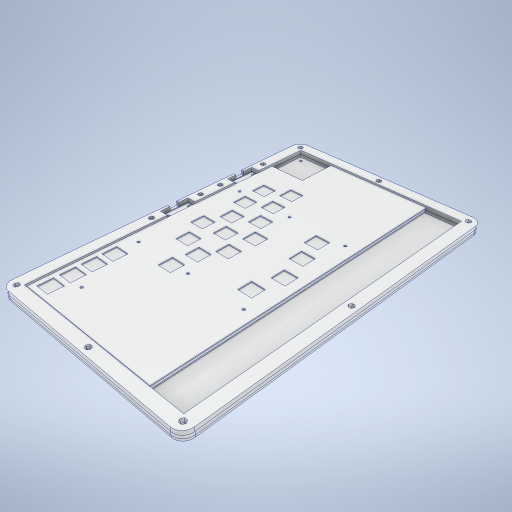
# Autodesk Inventor part: frame
Saved by Autodesk Inventor 2024 (Build 280153000, 153)
## iProperties
Created: 2023-10-23
Part Number: frame
Material: 铝 6061
Document SubType Name: Modeling
Designer: nicx5
Density: 2.7 g/cm^3
Appearance: 铝 - 平面
Author: nicx5
Autodesk Inventor part; units mm, degrees
ref_plane "YZ Plane" through (0, 0, 0) normal (1, 0, 0) x (0, 1, 0)
ref_plane "XY Plane" through (0, 0, 0) normal (0, 0, 1) x (1, 0, 0)
ref_plane "FloorFirst平面" through (0, 2, 0) normal (0, 1, 0) x (-1, 0, 0)
ref_plane "FloorSecond平面" through (0, 5, 0) normal (0, 1, 0) x (-1, 0, 0)
ref_plane "TopPlate平面" through (0, 9, 0) normal (0, 1, 0) x (-1, 0, 0)
ref_plane "PCB平面" through (0, 3.8, 0) normal (0, 1, 0) x (-1, 0, 0)
ref_plane "PositionPlate平面" through (0, 7, 0) normal (0, 1, 0) x (-1, 0, 0)
sketch "OLED草图" plane through (0, 0, 0) normal (0, 1, 0) x (-1, 0, 0)
  line L0 (84.9998, -145.0002) -> (84.9998, -109.6002)
  line L1 (84.9998, -109.6002) -> (51.4998, -109.6002)
  line L2 (51.4998, -145.0002) -> (84.9998, -145.0002)
  line L3 (51.4998, -109.6002) -> (51.4998, -145.0002)
  circle A0 centre (82.4998, -112.2002) radius 1.5
  circle A1 centre (82.4998, -142.4002) radius 1.5
  circle A2 centre (53.9998, -112.2002) radius 1.5
  circle A3 centre (53.9998, -142.4002) radius 1.5
  line L4 (61.9498, -111.5902) -> (61.9498, -143.0102)
  line L5 (61.9498, -143.0102) -> (78.6498, -143.0102)
  line L6 (78.6498, -143.0102) -> (78.6498, -111.5902)
  line L7 (78.6498, -111.5902) -> (61.9498, -111.5902)
  line L8 (84.9998, -115.8002) -> (78.6498, -115.8002)
  line L9 (78.6498, -115.8002) -> (78.6498, -138.8002)
  line L10 (78.6498, -138.8002) -> (84.9998, -138.8002)
  line L11 (84.9998, -138.8002) -> (84.9998, -115.8002)
  point P0 (0, 0)
  constraints: 24 end point, 4 centre point
sketch "BottomPlate草图" plane through (0, 0, 0) normal (0, 1, 0) x (-1, 0, 0)
  line L0 (90, 160) -> (-90, 160)
  line L1 (-100, 150) -> (-100, -150)
  line L2 (-90, -160) -> (90, -160)
  line L3 (100, -150) -> (100, 150)
  line L4 (-100, 160) -> (100, -160) construction
  circle A0 centre (92, 152) radius 1.6
  circle A1 centre (92, -152) radius 1.6
  circle A2 centre (-92, 152) radius 1.6
  circle A3 centre (-92, -152) radius 1.6
  arc A4 (100, 150) -> (90, 160) centre (90, 150) ccw
  arc A5 (-90, 160) -> (-100, 150) centre (-90, 150) ccw
  arc A6 (-100, -150) -> (-90, -160) centre (-90, -150) ccw
  arc A7 (90, -160) -> (100, -150) centre (90, -150) ccw
  circle A8 centre (94, 26.75) radius 2.75
  circle A9 centre (94, -26.75) radius 2.75
  circle A10 centre (94, -49.75) radius 2.75
  circle A11 centre (94, -103.25) radius 2.75
  circle A12 centre (0, 154) radius 2.75
  circle A13 centre (0, -153.5) radius 2.75
  circle A14 centre (-94, 0) radius 2.75
  circle A15 centre (91.5, 11) radius 1.35
  circle A16 centre (91.5, -11) radius 1.35
  circle A17 centre (91.5, -65.5) radius 1.35
  circle A18 centre (91.5, -87.5) radius 1.35
  circle A19 centre (16, 55) radius 1.35
  circle A20 centre (16, -55) radius 1.35
  circle A21 centre (75, 55) radius 1.35
  circle A22 centre (75, -55) radius 1.35
  circle A23 centre (57.5, 120) radius 1.35
  circle A24 centre (-43, 55) radius 1.35
  circle A25 centre (-43, -55) radius 1.35
  circle A26 centre (82.4998, -112.2002) radius 1.5 projected
  circle A27 centre (82.4998, -142.4002) radius 1.5 projected
  circle A28 centre (53.9998, -142.4002) radius 1.5 projected
  circle A29 centre (53.9998, -112.2002) radius 1.5 projected
  dimension "d12" = 3.2
  dimension "d13" = 3.2
  dimension "d14" = 3.2
  dimension "d15" = 3.2
  dimension "d16" = 10
  dimension "d58" = 5.5
  dimension "d59" = 5.5
  dimension "d60" = 5.5
  dimension "d61" = 5.5
  dimension "d63" = 5.5
  dimension "d65" = 5.5
  dimension "d67" = 5.5
  dimension "d210" = 2.7
  dimension "d211" = 2.7
  dimension "d214" = 2.7
  dimension "d215" = 2.7
  dimension "d218" = 2.7
  dimension "d219" = 2.7
  dimension "d227" = 2.7
  dimension "d228" = 2.7
  dimension "d237" = 2.7
  dimension "d325" = 2.7
  dimension "d326" = 2.7
  constraints: 26 centre point, 10 end point, 8 point on circle, 8 tangent, 4 point on line, 3 equal radius
  measures "d12" diameter of A0
  measures "d13" diameter of A1
  measures "d14" diameter of A2
  measures "d15" diameter of A3
  measures "d16" radius of A4
  measures "d58" diameter of A8
  measures "d59" diameter of A9
  measures "d60" diameter of A10
  measures "d61" diameter of A11
  measures "d63" diameter of A12
  measures "d65" diameter of A13
  measures "d67" diameter of A14
  measures "d210" diameter of A15
  measures "d211" diameter of A16
  measures "d214" diameter of A17
  measures "d215" diameter of A18
  measures "d218" diameter of A19
  measures "d219" diameter of A20
  measures "d227" diameter of A21
  measures "d228" diameter of A22
  measures "d237" diameter of A23
  measures "d325" diameter of A24
  measures "d326" diameter of A25
sketch "FloorFirst草图" plane through (0, 2, 0) normal (0, 1, 0) x (-1, 0, 0)
  arc A0 (100, 150) -> (90, 160) centre (90, 150) ccw
  line L0 (100, -150) -> (100, 150)
  arc A1 (90, -160) -> (100, -150) centre (90, -150) ccw
  line L1 (-90, -160) -> (90, -160)
  arc A2 (-100, -150) -> (-90, -160) centre (-90, -150) ccw
  line L2 (-100, 150) -> (-100, -150)
  arc A3 (-90, 160) -> (-100, 150) centre (-90, 150) ccw
  line L3 (90, 160) -> (-90, 160)
  circle A4 centre (-92, 152) radius 1.6
  line L4 (89.2557, 152) -> (90.6279, 154.3766)
  line L5 (90.6279, 154.3766) -> (93.3721, 154.3766)
  line L6 (93.3721, 154.3766) -> (94.7443, 152)
  line L7 (94.7443, 152) -> (93.3721, 149.6234)
  line L8 (93.3721, 149.6234) -> (90.6279, 149.6234)
  line L9 (90.6279, 149.6234) -> (89.2557, 152)
  line L10 (-94.7495, 152) -> (-93.3747, 154.3811)
  line L11 (-93.3747, 154.3811) -> (-90.6253, 154.3811)
  line L12 (-90.6253, 154.3811) -> (-89.2505, 152)
  line L13 (-89.2505, 152) -> (-90.6253, 149.6189)
  line L14 (-90.6253, 149.6189) -> (-93.3747, 149.6189)
  line L15 (-93.3747, 149.6189) -> (-94.7495, 152)
  line L16 (-94.7495, -152) -> (-93.3747, -149.6189)
  line L17 (-93.3747, -149.6189) -> (-90.6253, -149.6189)
  line L18 (-90.6253, -149.6189) -> (-89.2505, -152)
  line L19 (-89.2505, -152) -> (-90.6253, -154.3811)
  line L20 (-90.6253, -154.3811) -> (-93.3747, -154.3811)
  line L21 (-93.3747, -154.3811) -> (-94.7495, -152)
  line L22 (89.2506, -152) -> (90.6253, -149.6189)
  line L23 (90.6253, -149.6189) -> (93.3747, -149.6189)
  line L24 (93.3747, -149.6189) -> (94.7494, -152)
  line L25 (94.7494, -152) -> (93.3747, -154.3811)
  line L26 (93.3747, -154.3811) -> (90.6253, -154.3811)
  line L27 (90.6253, -154.3811) -> (89.2506, -152)
  line L28 (88, 148) -> (-88, 148)
  line L29 (-88, 148) -> (-88, -148)
  line L30 (-88, -148) -> (88, -148)
  line L31 (97, -15) -> (97, 15)
  line L32 (97, -15) -> (97, -4.9)
  line L33 (88, -15) -> (97, -15)
  line L34 (97, 15) -> (88, 15)
  line L35 (97, -61.5) -> (97, -91.5)
  line L36 (97, -81.4) -> (97, -91.5)
  line L37 (97, -91.5) -> (88, -91.5)
  line L38 (88, -61.5) -> (97, -61.5)
  line L39 (88, 15) -> (88, 148)
  line L40 (88, -148) -> (88, -91.5)
  line L41 (88, -61.5) -> (88, -15)
  line L42 (91.25, 26.75) -> (92.625, 29.1316)
  line L43 (92.625, 29.1316) -> (95.375, 29.1316)
  line L44 (95.375, 29.1316) -> (96.75, 26.75)
  line L45 (96.75, 26.75) -> (95.375, 24.3684)
  line L46 (95.375, 24.3684) -> (92.625, 24.3684)
  line L47 (92.625, 24.3684) -> (91.25, 26.75)
  line L48 (91.25, -26.75) -> (92.625, -24.3684)
  line L49 (92.625, -24.3684) -> (95.375, -24.3684)
  line L50 (95.375, -24.3684) -> (96.75, -26.75)
  line L51 (96.75, -26.75) -> (95.375, -29.1316)
  line L52 (95.375, -29.1316) -> (92.625, -29.1316)
  line L53 (92.625, -29.1316) -> (91.25, -26.75)
  line L54 (91.25, -49.75) -> (92.625, -47.3684)
  line L55 (92.625, -47.3684) -> (95.375, -47.3684)
  line L56 (95.375, -47.3684) -> (96.75, -49.75)
  line L57 (96.75, -49.75) -> (95.375, -52.1316)
  line L58 (95.375, -52.1316) -> (92.625, -52.1316)
  line L59 (92.625, -52.1316) -> (91.25, -49.75)
  line L60 (91.25, -103.25) -> (92.625, -100.8684)
  line L61 (92.625, -100.8684) -> (95.375, -100.8684)
  line L62 (95.375, -100.8684) -> (96.75, -103.25)
  line L63 (96.75, -103.25) -> (95.375, -105.6316)
  line L64 (95.375, -105.6316) -> (92.625, -105.6316)
  line L65 (92.625, -105.6316) -> (91.25, -103.25)
  line L66 (-2.7499, 154) -> (-1.375, 156.3815)
  line L67 (-1.375, 156.3815) -> (1.375, 156.3815)
  line L68 (1.375, 156.3815) -> (2.7499, 154)
  line L69 (2.7499, 154) -> (1.375, 151.6185)
  line L70 (1.375, 151.6185) -> (-1.375, 151.6185)
  line L71 (-1.375, 151.6185) -> (-2.7499, 154)
  line L72 (-2.7499, -153.5) -> (-1.375, -151.1185)
  line L73 (-1.375, -151.1185) -> (1.375, -151.1185)
  line L74 (1.375, -151.1185) -> (2.7499, -153.5)
  line L75 (2.7499, -153.5) -> (1.375, -155.8815)
  line L76 (1.375, -155.8815) -> (-1.375, -155.8815)
  line L77 (-1.375, -155.8815) -> (-2.7499, -153.5)
  line L78 (-96.75, 0) -> (-95.375, 2.3816)
  line L79 (-95.375, 2.3816) -> (-92.625, 2.3816)
  line L80 (-92.625, 2.3816) -> (-91.25, 0)
  line L81 (-91.25, 0) -> (-92.625, -2.3816)
  line L82 (-92.625, -2.3816) -> (-95.375, -2.3816)
  line L83 (-95.375, -2.3816) -> (-96.75, 0)
  point P0 (0, 0)
  point P1 (92, 152)
  point P2 (-92, -152)
  point P3 (92, -152)
  point P4 (94, 26.75)
  point P5 (94, -26.75)
  point P6 (94, -49.75)
  point P7 (94, -103.25)
  point P8 (0, 154)
  point P9 (0, -153.5)
  point P10 (-94, 0)
  constraints: 168 end point, 8 point on circle, 5 centre point, 145 other
sketch "FloorSecond草图" plane through (0, 5, 0) normal (0, 1, 0) x (-1, 0, 0)
  arc A0 (100, 150) -> (90, 160) centre (90, 150) ccw
  line L0 (90, 160) -> (-90, 160)
  arc A1 (-90, 160) -> (-100, 150) centre (-90, 150) ccw
  line L1 (-100, 150) -> (-100, -150)
  arc A2 (-100, -150) -> (-90, -160) centre (-90, -150) ccw
  line L2 (-90, -160) -> (90, -160)
  arc A3 (90, -160) -> (100, -150) centre (90, -150) ccw
  line L3 (88, 148) -> (-88, 148)
  line L4 (-88, 148) -> (-88, -148)
  line L5 (-88, -148) -> (88, -148)
  line L6 (94.7443, 152) -> (93.3721, 149.6234)
  line L7 (93.3721, 154.3766) -> (94.7443, 152)
  line L8 (90.6279, 154.3766) -> (93.3721, 154.3766)
  line L9 (89.2557, 152) -> (90.6279, 154.3766)
  line L10 (90.6279, 149.6234) -> (89.2557, 152)
  line L11 (93.3721, 149.6234) -> (90.6279, 149.6234)
  line L12 (90.6253, -149.6189) -> (93.3747, -149.6189)
  line L13 (93.3747, -149.6189) -> (94.7494, -152)
  line L14 (94.7494, -152) -> (93.3747, -154.3811)
  line L15 (93.3747, -154.3811) -> (90.6253, -154.3811)
  line L16 (90.6253, -154.3811) -> (89.2506, -152)
  line L17 (89.2506, -152) -> (90.6253, -149.6189)
  line L18 (-89.2505, -152) -> (-90.6253, -154.3811)
  line L19 (-90.6253, -149.6189) -> (-89.2505, -152)
  line L20 (-93.3747, -149.6189) -> (-90.6253, -149.6189)
  line L21 (-94.7495, -152) -> (-93.3747, -149.6189)
  line L22 (-93.3747, -154.3811) -> (-94.7495, -152)
  line L23 (-90.6253, -154.3811) -> (-93.3747, -154.3811)
  line L24 (-90.6253, 154.3811) -> (-89.2505, 152)
  line L25 (-93.3747, 154.3811) -> (-90.6253, 154.3811)
  line L26 (-94.7495, 152) -> (-93.3747, 154.3811)
  line L27 (-93.3747, 149.6189) -> (-94.7495, 152)
  line L28 (-90.6253, 149.6189) -> (-93.3747, 149.6189)
  line L29 (-89.2505, 152) -> (-90.6253, 149.6189)
  line L30 (97, 15) -> (88, 15)
  line L31 (88, -15) -> (97, -15)
  line L32 (88, 15) -> (88, 148)
  line L33 (100, 4.9) -> (97, 4.9)
  line L34 (97, -4.9) -> (100, -4.9)
  line L35 (97, -15) -> (97, -4.9)
  line L36 (97, 4.9) -> (97, 15)
  line L37 (88, -15) -> (93, -15)
  line L38 (93, -61.5) -> (88, -61.5)
  line L39 (88, -61.5) -> (88, -15)
  line L40 (88, -61.5) -> (97, -61.5)
  line L41 (97, -91.5) -> (88, -91.5)
  line L42 (100, -71.6) -> (97, -71.6)
  line L43 (97, -81.4) -> (100, -81.4)
  line L44 (97, -61.5) -> (97, -71.6)
  line L45 (97, -81.4) -> (97, -91.5)
  line L46 (100, 4.9) -> (100, 150)
  line L47 (100, -150) -> (100, -81.4)
  line L48 (100, -71.6) -> (100, -4.9)
  line L49 (88, -148) -> (88, -91.5)
  line L50 (88, -61.5) -> (88, -15)
  line L51 (96.75, 26.75) -> (95.375, 24.3684)
  line L52 (95.375, 29.1316) -> (96.75, 26.75)
  line L53 (92.625, 29.1316) -> (95.375, 29.1316)
  line L54 (91.25, 26.75) -> (92.625, 29.1316)
  line L55 (92.625, 24.3684) -> (91.25, 26.75)
  line L56 (95.375, 24.3684) -> (92.625, 24.3684)
  line L57 (96.75, -26.75) -> (95.375, -29.1316)
  line L58 (95.375, -24.3684) -> (96.75, -26.75)
  line L59 (92.625, -24.3684) -> (95.375, -24.3684)
  line L60 (91.25, -26.75) -> (92.625, -24.3684)
  line L61 (92.625, -29.1316) -> (91.25, -26.75)
  line L62 (95.375, -29.1316) -> (92.625, -29.1316)
  line L63 (95.375, -47.3684) -> (96.75, -49.75)
  line L64 (92.625, -47.3684) -> (95.375, -47.3684)
  line L65 (91.25, -49.75) -> (92.625, -47.3684)
  line L66 (92.625, -52.1316) -> (91.25, -49.75)
  line L67 (95.375, -52.1316) -> (92.625, -52.1316)
  line L68 (96.75, -49.75) -> (95.375, -52.1316)
  line L69 (95.375, -100.8684) -> (96.75, -103.25)
  line L70 (92.625, -100.8684) -> (95.375, -100.8684)
  line L71 (91.25, -103.25) -> (92.625, -100.8684)
  line L72 (92.625, -105.6316) -> (91.25, -103.25)
  line L73 (95.375, -105.6316) -> (92.625, -105.6316)
  line L74 (96.75, -103.25) -> (95.375, -105.6316)
  line L75 (2.7499, -153.5) -> (1.375, -155.8815)
  line L76 (1.375, -151.1185) -> (2.7499, -153.5)
  line L77 (-1.375, -151.1185) -> (1.375, -151.1185)
  line L78 (-2.7499, -153.5) -> (-1.375, -151.1185)
  line L79 (-1.375, -155.8815) -> (-2.7499, -153.5)
  line L80 (1.375, -155.8815) -> (-1.375, -155.8815)
  line L81 (-91.25, 0) -> (-92.625, -2.3816)
  line L82 (-92.625, 2.3816) -> (-91.25, 0)
  line L83 (-95.375, 2.3816) -> (-92.625, 2.3816)
  line L84 (-96.75, 0) -> (-95.375, 2.3816)
  line L85 (-95.375, -2.3816) -> (-96.75, 0)
  line L86 (-92.625, -2.3816) -> (-95.375, -2.3816)
  line L87 (1.375, 156.3815) -> (2.7499, 154)
  line L88 (-1.375, 156.3815) -> (1.375, 156.3815)
  line L89 (-2.7499, 154) -> (-1.375, 156.3815)
  line L90 (-1.375, 151.6185) -> (-2.7499, 154)
  line L91 (1.375, 151.6185) -> (-1.375, 151.6185)
  line L92 (2.7499, 154) -> (1.375, 151.6185)
  point P0 (0, 0)
  point P1 (88, 0)
  point P2 (97, 0)
  point P3 (97, -76.5)
  constraints: 186 end point, 8 point on circle, 4 centre point
sketch "TopPlate草图" plane through (0, 9, 0) normal (0, 1, 0) x (-1, 0, 0)
  line L0 (100, 4.9) -> (100, 150)
  arc A0 (100, 150) -> (90, 160) centre (90, 150) ccw
  line L1 (90, 160) -> (-90, 160)
  line L2 (100, -150) -> (100, 150)
  arc A1 (90, -160) -> (100, -150) centre (90, -150) ccw
  line L3 (-90, -160) -> (90, -160)
  arc A2 (-100, -150) -> (-90, -160) centre (-90, -150) ccw
  line L4 (-100, 150) -> (-100, -150)
  arc A3 (-90, 160) -> (-100, 150) centre (-90, 150) ccw
  circle A4 centre (92, 152) radius 1.6
  circle A5 centre (92, -152) radius 1.6
  circle A6 centre (-92, -152) radius 1.6
  circle A7 centre (-92, 152) radius 1.6
  line L5 (32.0321, 53.8512) -> (32.0321, 31.8512) construction
  arc A8 (15.4226, 25.1627) -> (25.9869, 17.7656) centre (15.5932, 14.1641) ccw
  line L6 (28.2118, 32.1854) -> (28.2118, 10.1854) construction
  circle A9 centre (13.4288, -12.5738) radius 11
  circle A10 centre (-30.7795, 35.3233) radius 11
  line L7 (-30.7795, 35.3233) -> (-37.9769, 8.2642)
  line L8 (-37.9769, 8.2642) -> (-30.7795, -18.795)
  circle A11 centre (-37.9769, 8.2642) radius 13.5
  circle A12 centre (-30.7795, -18.795) radius 11
  line L9 (13.4288, -12.5738) -> (-10.8955, -12.5738) construction
  line L10 (13.4288, -12.5738) -> (-18.1395, -12.5738) construction
  line L11 (13.4288, -12.5738) -> (-18.1395, -12.5738) construction
  line L12 (13.4288, -12.5738) -> (27.7683, -33.0526)
  line L13 (13.4288, -12.5738) -> (-11.5712, -12.5738) construction
  line L14 (27.7683, -33.0526) -> (36.3188, -56.5449)
  line L15 (36.3188, -56.5449) -> (38.4977, -81.4497)
  line L16 (15.5932, 14.1641) -> (29.0722, 33.4141)
  line L17 (15.5932, 14.1641) -> (-7.9068, 14.1641) construction
  line L18 (29.0722, 33.4141) -> (33.1529, 56.5571)
  circle A13 centre (27.7683, -33.0526) radius 11
  circle A14 centre (36.3188, -56.5449) radius 11
  circle A15 centre (38.4977, -81.4497) radius 11
  line L19 (58.7471, -45.803) -> (60.926, -70.7079)
  circle A16 centre (60.926, -70.7079) radius 11
  circle A17 centre (58.7471, -45.803) radius 11
  circle A18 centre (35.8572, -1.8319) radius 11
  circle A19 centre (50.1966, -22.3107) radius 11
  line L20 (50.1966, -22.3107) -> (58.7471, -45.803)
  line L21 (35.8572, -1.8319) -> (50.1966, -22.3107)
  circle A20 centre (60.7621, 0.347) radius 11
  line L22 (-30.7795, -18.795) -> (-24.4131, -42.9707)
  circle A21 centre (-24.4131, -42.9707) radius 11
  line L23 (36.0371, 44.12) -> (36.0361, 44.1148)
  line L24 (26.43, 20.9234) -> (26.4269, 20.919)
  line L25 (26.189, 45.8565) -> (26.1881, 45.8512)
  line L26 (18.2384, 26.6592) -> (18.2354, 26.6548)
  arc A22 (37.9557, 46.661) -> (25.2551, 48.9005) centre (33.1529, 56.5571) ccw
  arc A23 (24.2694, 43.3102) -> (18.6785, 29.8126) centre (29.0722, 33.4141) ccw
  arc A24 (37.9557, 46.661) -> (36.0371, 44.12) centre (39.4839, 43.5122) ccw
  arc A25 (36.0361, 44.1148) -> (36.97, 41.0708) centre (39.483, 43.507) ccw
  arc A26 (26.189, 45.8565) -> (25.2551, 48.9005) centre (22.7422, 46.4642) ccw
  arc A27 (24.2694, 43.3102) -> (26.1881, 45.8512) centre (22.7412, 46.459) ccw
  arc A28 (29.2427, 22.4155) -> (26.43, 20.9234) centre (29.297, 18.9159) ccw
  arc A29 (26.4269, 20.919) -> (25.9869, 17.7656) centre (29.2939, 18.9115) ccw
  arc A30 (18.2384, 26.6592) -> (18.6785, 29.8126) centre (15.3714, 28.6667) ccw
  arc A31 (15.4226, 25.1627) -> (18.2354, 26.6548) centre (15.3684, 28.6623) ccw
  line L27 (85, 145) -> (64.7, 145)
  line L28 (64.7, 145) -> (64.7, 67.7)
  line L29 (64.7, 67.7) -> (85, 67.7)
  line L30 (85, 67.7) -> (85, 145)
  line L31 (74.85, 134.85) -> (74.85, 115.85)
  line L32 (74.85, 115.85) -> (74.85, 96.85)
  line L33 (74.85, 96.85) -> (74.85, 77.85)
  line L34 (29.0722, 33.4141) -> (50.7834, 24.4211)
  line L35 (29.0722, 33.4141) -> (52.5722, 33.4141) construction
  arc A32 (40.0823, 21.874) -> (45.0176, 33.7889) centre (50.7834, 24.4211) ccw
  arc A33 (29.2427, 22.4155) -> (34.838, 24.0463) centre (29.0722, 33.4141) ccw
  arc A34 (39.7733, 35.9612) -> (36.97, 41.0708) centre (29.0722, 33.4141) ccw
  line L36 (38.0168, 24.2972) -> (38.0119, 24.2992)
  line L37 (41.8437, 33.536) -> (41.8387, 33.538)
  arc A35 (40.0823, 21.874) -> (38.0168, 24.2972) centre (36.6774, 21.0636) ccw
  arc A36 (38.0119, 24.2992) -> (34.838, 24.0463) centre (36.6725, 21.0656) ccw
  arc A37 (41.8437, 33.536) -> (45.0176, 33.7889) centre (43.1831, 36.7696) ccw
  arc A38 (39.7733, 35.9612) -> (41.8387, 33.538) centre (43.1781, 36.7716) ccw
  line L38 (84.9998, -109.6002) -> (51.4998, -109.6002)
  line L39 (51.4998, -109.6002) -> (51.4998, -145.0002)
  line L40 (51.4998, -145.0002) -> (84.9998, -145.0002)
  line L41 (84.9998, -145.0002) -> (84.9998, -109.6002)
  line L42 (84.9998, -115.8002) -> (78.6498, -115.8002)
  line L43 (78.6498, -115.8002) -> (78.6498, -138.8002)
  line L44 (78.6498, -138.8002) -> (84.9998, -138.8002)
  line L45 (84.9998, -138.8002) -> (84.9998, -115.8002)
  line L46 (78.6498, -111.5902) -> (61.9498, -111.5902)
  line L47 (61.9498, -111.5902) -> (61.9498, -143.0102)
  line L48 (61.9498, -143.0102) -> (78.6498, -143.0102)
  line L49 (78.6498, -143.0102) -> (78.6498, -111.5902)
  line L50 (84.9998, -109.6002) -> (82.4998, -109.6002)
  line L51 (82.4998, -109.6002) -> (82.4998, -112.2002)
  line L52 (82.4998, -112.2002) -> (84.9998, -112.2002)
  line L53 (84.9998, -112.2002) -> (84.9998, -109.6002)
  line L54 (84.9998, -145.0002) -> (82.4998, -145.0002)
  line L55 (82.4998, -145.0002) -> (82.4998, -142.4002)
  line L56 (82.4998, -142.4002) -> (84.9998, -142.4002)
  line L57 (84.9998, -142.4002) -> (84.9998, -145.0002)
  line L58 (51.4998, -109.6002) -> (53.9998, -109.6002)
  line L59 (53.9998, -109.6002) -> (53.9998, -112.2002)
  line L60 (53.9998, -112.2002) -> (51.4998, -112.2002)
  line L61 (51.4998, -112.2002) -> (51.4998, -109.6002)
  line L62 (51.4998, -145.0002) -> (53.9998, -145.0002)
  line L63 (53.9998, -145.0002) -> (53.9998, -142.4002)
  line L64 (53.9998, -142.4002) -> (51.4998, -142.4002)
  line L65 (51.4998, -142.4002) -> (51.4998, -145.0002)
  circle A39 centre (82.4998, -112.2002) radius 1.5
  circle A40 centre (82.4998, -142.4002) radius 1.5
  circle A41 centre (53.9998, -142.4002) radius 1.5
  circle A42 centre (53.9998, -112.2002) radius 1.5
  circle A43 centre (92, 152) radius 1.6 projected
  circle A44 centre (0, 154) radius 2.75 projected
  circle A45 centre (-92, 152) radius 1.6 projected
  circle A46 centre (-94, 0) radius 2.75 projected
  circle A47 centre (-92, -152) radius 1.6 projected
  circle A48 centre (0, -153.5) radius 2.75 projected
  circle A49 centre (92, -152) radius 1.6 projected
  circle A50 centre (94, 26.75) radius 2.75 projected
  circle A51 centre (94, -26.75) radius 2.75 projected
  point P0 (33.9026, 43.7117)
  point P1 (36.3756, 46.0398)
  point P2 (27.5481, 22.5202)
  point P3 (26.5275, 47.7762)
  point P4 (17.1173, 25.058)
  point P5 (35.6976, 42.195)
  point P6 (25.8496, 43.9315)
  point P7 (19.3566, 28.256)
  point P8 (25.3088, 19.3222)
  point P9 (39.8178, 23.5512)
  point P10 (43.6447, 32.79)
  point P11 (36.2109, 25.0452)
  point P12 (40.0378, 34.284)
  dimension "d102" = 22
  dimension "d103" = 22
  dimension "d104" = 27
  dimension "d105" = 22
  dimension "d106" = 22
  dimension "d107" = 25
  dimension "d108" = 125
  dimension "d109" = 25
  dimension "d110" = 165
  dimension "d111" = 25
  dimension "d112" = 165
  dimension "d113" = 23.5
  dimension "d114" = 125
  dimension "d115" = 23.5
  dimension "d116" = 155
  dimension "d117" = 22
  dimension "d118" = 22
  dimension "d119" = 22
  dimension "d120" = 22
  dimension "d121" = 25
  dimension "d122" = 25
  dimension "d123" = 165
  dimension "d124" = 25
  dimension "d125" = 165
  dimension "d126" = 22
  dimension "d127" = 22
  dimension "d128" = 22
  dimension "d129" = 22
  dimension "d130" = 25
  dimension "d131" = 22
  dimension "d134" = 5
  dimension "d135" = 5
  dimension "d136" = 3.5
  dimension "d137" = 3.5
  dimension "d138" = 3.5
  dimension "d139" = 3.5
  dimension "d142" = 20.3
  dimension "d143" = 77.3
  dimension "d145" = 19
  dimension "d146" = 19
  dimension "d147" = 19
  dimension "d169" = 23.5
  dimension "d170" = 22.5
  dimension "d171" = 22
  dimension "d174" = 3.5
  dimension "d175" = 3.5
  dimension "d180" = 33.5
  dimension "d181" = 35.4
  dimension "d183" = 6.35
  dimension "d184" = 23
  dimension "d186" = 16.7
  dimension "d187" = 31.42
  dimension "d188" = 2.5
  dimension "d189" = 2.6
  dimension "d190" = 2.5
  dimension "d191" = 2.6
  dimension "d192" = 2.5
  dimension "d193" = 2.6
  dimension "d194" = 2.5
  dimension "d195" = 2.6
  dimension "d196" = 3
  dimension "d197" = 3
  dimension "d198" = 3
  dimension "d199" = 3
  constraints: 132 end point, 54 point on circle, 43 centre point, 22 tangent, 13 point on line, 8 coincident, 6 equal radius, 3 equal length, 1 horizontal, 1 parallel
  measures "d102" diameter of A8
  measures "d103" diameter of A9
  measures "d104" diameter of A11
  measures "d105" diameter of A10
  measures "d106" diameter of A12
  measures "d107" distance of L12.start L12.end
  measures "d108" angle of L13 L12
  measures "d109" distance of L12.end L14.end
  measures "d110" angle of L12 L14
  measures "d111" distance of L14.end L15.end
  measures "d112" angle of L14 L15
  measures "d113" distance of L16.start L16.end
  measures "d114" angle of L16 L17
  measures "d115" distance of L16.end L18.end
  measures "d116" angle of L18 L16
  measures "d117" diameter of A13
  measures "d118" diameter of A14
  measures "d119" diameter of A15
  measures "d120" diameter of A18
  measures "d121" distance of L21.start L21.end
  measures "d122" distance of L21.end L20.end
  measures "d123" angle of L21 L20
  measures "d124" distance of L20.end L19.end
  measures "d125" angle of L20 L19
  measures "d126" diameter of A19
  measures "d127" diameter of A17
  measures "d128" diameter of A16
  measures "d129" diameter of A20
  measures "d130" distance of L22.start L22.end
  measures "d131" diameter of A21
  measures "d134" distance between parallel lines of L18 L23
  measures "d135" distance between parallel lines of L18 L25
  measures "d136" radius of A24
  measures "d137" radius of A26
  measures "d138" radius of A27
  measures "d139" radius of A28
  measures "d142" distance of L29.end L28.end
  measures "d143" distance of L28.end L27.end
  measures "d145" distance of L31.start L31.end
  measures "d146" distance of L32.start L32.end
  measures "d147" distance of L33.start L33.end
  measures "d169" distance of L34.start L34.end
  measures "d170" angle of L34 L35
  measures "d171" diameter of A32
  measures "d174" radius of A35
  measures "d175" radius of A37
  measures "d180" distance of L40.end L39.end
  measures "d181" distance of L39.end L38.end
  measures "d183" distance of L44.end L43.end
  measures "d184" distance of L43.end L42.end
  measures "d186" distance of L48.end L47.end
  measures "d187" distance of L47.end L46.end
  measures "d188" distance of L52.end L51.end
  measures "d189" distance of L51.end L50.end
  measures "d190" distance of L55.end L56.end
  measures "d191" distance of L54.end L55.end
  measures "d192" distance of L59.end L60.end
  measures "d193" distance of L58.end L59.end
  measures "d194" distance of L64.end L63.end
  measures "d195" distance of L63.end L62.end
  measures "d196" diameter of A39
  measures "d197" diameter of A40
  measures "d198" diameter of A41
  measures "d199" diameter of A42
sketch "PositionPlate草图" plane through (0, 7, 0) normal (0, 1, 0) x (-1, 0, 0)
  line L0 (87, 147) -> (87, -107.6002)
  line L1 (87, -90.5) -> (87, -147)
  line L2 (49.4998, -147) -> (-54.9998, -147)
  line L3 (-54.9998, -147) -> (-54.9998, 147)
  line L4 (-54.9998, 147) -> (87, 147)
  line L5 (74.85, 134.85) -> (74.85, 115.85) projected
  line L6 (74.85, 115.85) -> (74.85, 96.85) projected
  line L7 (74.85, 96.85) -> (74.85, 77.85) projected
  line L8 (29.0722, 33.4141) -> (50.7834, 24.4211) projected
  line L9 (29.0722, 33.4141) -> (33.1529, 56.5571) projected
  line L10 (15.5932, 14.1641) -> (29.0722, 33.4141) projected
  line L11 (35.8572, -1.8319) -> (50.1966, -22.3107) projected
  line L12 (50.1966, -22.3107) -> (58.7471, -45.803) projected
  line L13 (58.7471, -45.803) -> (60.926, -70.7079) projected
  line L14 (13.4288, -12.5738) -> (27.7683, -33.0526) projected
  line L15 (27.7683, -33.0526) -> (36.3188, -56.5449) projected
  line L16 (36.3188, -56.5449) -> (38.4977, -81.4497) projected
  line L17 (-30.7795, 35.3233) -> (-37.9769, 8.2642) projected
  line L18 (-37.9769, 8.2642) -> (-30.7795, -18.795) projected
  line L19 (-30.7795, -18.795) -> (-24.4131, -42.9707) projected
  line L20 (81.875, 141.875) -> (67.825, 141.875)
  line L21 (67.825, 141.875) -> (67.825, 127.825)
  line L22 (67.825, 127.825) -> (81.875, 127.825)
  line L23 (81.875, 127.825) -> (81.875, 141.875)
  line L24 (81.875, 141.875) -> (67.825, 127.825) construction
  line L25 (67.825, 141.875) -> (81.875, 127.825) construction
  line L26 (81.875, 122.875) -> (67.825, 122.875)
  line L27 (67.825, 122.875) -> (67.825, 108.825)
  line L28 (67.825, 108.825) -> (81.875, 108.825)
  line L29 (81.875, 108.825) -> (81.875, 122.875)
  line L30 (81.875, 122.875) -> (67.825, 108.825) construction
  line L31 (67.825, 122.875) -> (81.875, 108.825) construction
  line L32 (81.875, 103.875) -> (67.825, 103.875)
  line L33 (67.825, 103.875) -> (67.825, 89.825)
  line L34 (67.825, 89.825) -> (81.875, 89.825)
  line L35 (81.875, 89.825) -> (81.875, 103.875)
  line L36 (81.875, 103.875) -> (67.825, 89.825) construction
  line L37 (67.825, 103.875) -> (81.875, 89.825) construction
  line L38 (81.875, 84.875) -> (67.825, 84.875)
  line L39 (67.825, 84.875) -> (67.825, 70.825)
  line L40 (67.825, 70.825) -> (81.875, 70.825)
  line L41 (81.875, 70.825) -> (81.875, 84.875)
  line L42 (81.875, 84.875) -> (67.825, 70.825) construction
  line L43 (67.825, 84.875) -> (81.875, 70.825) construction
  line L44 (40.1779, 63.5821) -> (26.1279, 63.5821)
  line L45 (26.1279, 63.5821) -> (26.1279, 49.5321)
  line L46 (26.1279, 49.5321) -> (40.1779, 49.5321)
  line L47 (40.1779, 49.5321) -> (40.1779, 63.5821)
  line L48 (40.1779, 63.5821) -> (26.1279, 49.5321) construction
  line L49 (26.1279, 63.5821) -> (40.1779, 49.5321) construction
  line L50 (57.8084, 31.4461) -> (43.7584, 31.4461)
  line L51 (43.7584, 31.4461) -> (43.7584, 17.3961)
  line L52 (43.7584, 17.3961) -> (57.8084, 17.3961)
  line L53 (57.8084, 17.3961) -> (57.8084, 31.4461)
  line L54 (57.8084, 31.4461) -> (43.7584, 17.3961) construction
  line L55 (43.7584, 31.4461) -> (57.8084, 17.3961) construction
  line L56 (36.0972, 40.4391) -> (22.0472, 40.4391)
  line L57 (22.0472, 40.4391) -> (22.0472, 26.3891)
  line L58 (22.0472, 26.3891) -> (36.0972, 26.3891)
  line L59 (36.0972, 26.3891) -> (36.0972, 40.4391)
  line L60 (36.0972, 40.4391) -> (22.0472, 26.3891) construction
  line L61 (22.0472, 40.4391) -> (36.0972, 26.3891) construction
  line L62 (22.6182, 21.1891) -> (8.5682, 21.1891)
  line L63 (8.5682, 21.1891) -> (8.5682, 7.1391)
  line L64 (8.5682, 7.1391) -> (22.6182, 7.1391)
  line L65 (22.6182, 7.1391) -> (22.6182, 21.1891)
  line L66 (22.6182, 21.1891) -> (8.5682, 7.1391) construction
  line L67 (8.5682, 21.1891) -> (22.6182, 7.1391) construction
  line L68 (42.8822, 5.1931) -> (28.8322, 5.1931)
  line L69 (28.8322, 5.1931) -> (28.8322, -8.8569)
  line L70 (28.8322, -8.8569) -> (42.8822, -8.8569)
  line L71 (42.8822, -8.8569) -> (42.8822, 5.1931)
  line L72 (42.8822, 5.1931) -> (28.8322, -8.8569) construction
  line L73 (28.8322, 5.1931) -> (42.8822, -8.8569) construction
  line L74 (20.4538, -5.5488) -> (6.4038, -5.5488)
  line L75 (6.4038, -5.5488) -> (6.4038, -19.5988)
  line L76 (6.4038, -19.5988) -> (20.4538, -19.5988)
  line L77 (20.4538, -19.5988) -> (20.4538, -5.5488)
  line L78 (20.4538, -5.5488) -> (6.4038, -19.5988) construction
  line L79 (6.4038, -5.5488) -> (20.4538, -19.5988) construction
  line L80 (34.7933, -26.0276) -> (20.7433, -26.0276)
  line L81 (20.7433, -26.0276) -> (20.7433, -40.0776)
  line L82 (20.7433, -40.0776) -> (34.7933, -40.0776)
  line L83 (34.7933, -40.0776) -> (34.7933, -26.0276)
  line L84 (34.7933, -26.0276) -> (20.7433, -40.0776) construction
  line L85 (20.7433, -26.0276) -> (34.7933, -40.0776) construction
  line L86 (43.3438, -49.5199) -> (29.2938, -49.5199)
  line L87 (29.2938, -49.5199) -> (29.2938, -63.5699)
  line L88 (29.2938, -63.5699) -> (43.3438, -63.5699)
  line L89 (43.3438, -63.5699) -> (43.3438, -49.5199)
  line L90 (43.3438, -49.5199) -> (29.2938, -63.5699) construction
  line L91 (29.2938, -49.5199) -> (43.3438, -63.5699) construction
  line L92 (45.5227, -74.4247) -> (31.4727, -74.4247)
  line L93 (31.4727, -74.4247) -> (31.4727, -88.4747)
  line L94 (31.4727, -88.4747) -> (45.5227, -88.4747)
  line L95 (45.5227, -88.4747) -> (45.5227, -74.4247)
  line L96 (45.5227, -74.4247) -> (31.4727, -88.4747) construction
  line L97 (31.4727, -74.4247) -> (45.5227, -88.4747) construction
  line L98 (57.2216, -15.2857) -> (43.1716, -15.2857)
  line L99 (43.1716, -15.2857) -> (43.1716, -29.3357)
  line L100 (43.1716, -29.3357) -> (57.2216, -29.3357)
  line L101 (57.2216, -29.3357) -> (57.2216, -15.2857)
  line L102 (57.2216, -15.2857) -> (43.1716, -29.3357) construction
  line L103 (43.1716, -15.2857) -> (57.2216, -29.3357) construction
  line L104 (65.7721, -38.778) -> (51.7221, -38.778)
  line L105 (51.7221, -38.778) -> (51.7221, -52.828)
  line L106 (51.7221, -52.828) -> (65.7721, -52.828)
  line L107 (65.7721, -52.828) -> (65.7721, -38.778)
  line L108 (65.7721, -38.778) -> (51.7221, -52.828) construction
  line L109 (51.7221, -38.778) -> (65.7721, -52.828) construction
  line L110 (67.951, -63.6829) -> (53.901, -63.6829)
  line L111 (53.901, -63.6829) -> (53.901, -77.7329)
  line L112 (53.901, -77.7329) -> (67.951, -77.7329)
  line L113 (67.951, -77.7329) -> (67.951, -63.6829)
  line L114 (67.951, -63.6829) -> (53.901, -77.7329) construction
  line L115 (53.901, -63.6829) -> (67.951, -77.7329) construction
  line L116 (67.7871, 7.372) -> (53.7371, 7.372)
  line L117 (53.7371, 7.372) -> (53.7371, -6.678)
  line L118 (53.7371, -6.678) -> (67.7871, -6.678)
  line L119 (67.7871, -6.678) -> (67.7871, 7.372)
  line L120 (67.7871, 7.372) -> (53.7371, -6.678) construction
  line L121 (53.7371, 7.372) -> (67.7871, -6.678) construction
  line L122 (-23.7545, 42.3483) -> (-37.8045, 42.3483)
  line L123 (-37.8045, 42.3483) -> (-37.8045, 28.2983)
  line L124 (-37.8045, 28.2983) -> (-23.7545, 28.2983)
  line L125 (-23.7545, 28.2983) -> (-23.7545, 42.3483)
  line L126 (-23.7545, 42.3483) -> (-37.8045, 28.2983) construction
  line L127 (-37.8045, 42.3483) -> (-23.7545, 28.2983) construction
  line L128 (-30.9519, 15.2892) -> (-45.0019, 15.2892)
  line L129 (-45.0019, 15.2892) -> (-45.0019, 1.2392)
  line L130 (-45.0019, 1.2392) -> (-30.9519, 1.2392)
  line L131 (-30.9519, 1.2392) -> (-30.9519, 15.2892)
  line L132 (-30.9519, 15.2892) -> (-45.0019, 1.2392) construction
  line L133 (-45.0019, 15.2892) -> (-30.9519, 1.2392) construction
  line L134 (-23.7545, -11.77) -> (-37.8045, -11.77)
  line L135 (-37.8045, -11.77) -> (-37.8045, -25.82)
  line L136 (-37.8045, -25.82) -> (-23.7545, -25.82)
  line L137 (-23.7545, -25.82) -> (-23.7545, -11.77)
  line L138 (-23.7545, -11.77) -> (-37.8045, -25.82) construction
  line L139 (-37.8045, -11.77) -> (-23.7545, -25.82) construction
  line L140 (-17.3881, -35.9457) -> (-31.4381, -35.9457)
  line L141 (-31.4381, -35.9457) -> (-31.4381, -49.9957)
  line L142 (-31.4381, -49.9957) -> (-17.3881, -49.9957)
  line L143 (-17.3881, -49.9957) -> (-17.3881, -35.9457)
  line L144 (-17.3881, -35.9457) -> (-31.4381, -49.9957) construction
  line L145 (-31.4381, -35.9457) -> (-17.3881, -49.9957) construction
  line L146 (84.9998, -109.6002) -> (51.4998, -109.6002) projected
  line L147 (51.4998, -109.6002) -> (51.4998, -145.0002) projected
  line L148 (87, -107.6002) -> (49.4998, -107.6002)
  line L149 (49.4998, -107.6002) -> (49.4998, -147)
  point P0 (0, 0)
  point P1 (60.7621, 0.347)
  dimension "d251" = 14.05
  dimension "d252" = 14.05
  dimension "d253" = 14.05
  dimension "d254" = 14.05
  dimension "d255" = 14.05
  dimension "d256" = 14.05
  dimension "d257" = 14.05
  dimension "d258" = 14.05
  dimension "d259" = 14.05
  dimension "d260" = 14.05
  dimension "d261" = 14.05
  dimension "d262" = 14.05
  dimension "d263" = 14.05
  dimension "d264" = 14.05
  dimension "d265" = 14.05
  dimension "d266" = 14.05
  dimension "d267" = 14.05
  dimension "d268" = 14.05
  dimension "d269" = 14.05
  dimension "d270" = 14.05
  dimension "d271" = 14.05
  dimension "d272" = 14.05
  dimension "d273" = 14.05
  dimension "d274" = 14.05
  dimension "d275" = 14.05
  dimension "d276" = 14.05
  dimension "d277" = 14.05
  dimension "d278" = 14.05
  dimension "d279" = 14.05
  dimension "d280" = 14.05
  dimension "d281" = 14.05
  dimension "d282" = 14.05
  dimension "d283" = 14.05
  dimension "d284" = 14.05
  dimension "d285" = 14.05
  dimension "d286" = 14.05
  dimension "d287" = 14.05
  dimension "d288" = 14.05
  dimension "d289" = 14.05
  dimension "d290" = 14.05
  dimension "d291" = 14.05
  dimension "d292" = 14.05
  dimension "d324" = 2
  constraints: 266 end point, 42 midpoint, 1 point on line
  measures "d251" distance of L22.end L21.end
  measures "d252" distance of L21.end L20.end
  measures "d253" distance of L28.end L27.end
  measures "d254" distance of L27.end L26.end
  measures "d255" distance of L34.end L33.end
  measures "d256" distance of L33.end L32.end
  measures "d257" distance of L40.end L39.end
  measures "d258" distance of L39.end L38.end
  measures "d259" distance of L46.end L45.end
  measures "d260" distance of L45.end L44.end
  measures "d261" distance of L52.end L51.end
  measures "d262" distance of L51.end L50.end
  measures "d263" distance of L58.end L57.end
  measures "d264" distance of L57.end L56.end
  measures "d265" distance of L64.end L63.end
  measures "d266" distance of L63.end L62.end
  measures "d267" distance of L70.end L69.end
  measures "d268" distance of L69.end L68.end
  measures "d269" distance of L76.end L75.end
  measures "d270" distance of L75.end L74.end
  measures "d271" distance of L82.end L81.end
  measures "d272" distance of L81.end L80.end
  measures "d273" distance of L88.end L87.end
  measures "d274" distance of L87.end L86.end
  measures "d275" distance of L94.end L93.end
  measures "d276" distance of L93.end L92.end
  measures "d277" distance of L100.end L99.end
  measures "d278" distance of L99.end L98.end
  measures "d279" distance of L106.end L105.end
  measures "d280" distance of L105.end L104.end
  measures "d281" distance of L112.end L111.end
  measures "d282" distance of L111.end L110.end
  measures "d283" distance of L118.end L117.end
  measures "d284" distance of L117.end L116.end
  measures "d285" distance of L124.end L123.end
  measures "d286" distance of L123.end L122.end
  measures "d287" distance of L130.end L129.end
  measures "d288" distance of L129.end L128.end
  measures "d289" distance of L136.end L135.end
  measures "d290" distance of L135.end L134.end
  measures "d291" distance of L142.end L141.end
  measures "d292" distance of L141.end L140.end
  measures "d324" distance between parallel lines of L146 L148
sketch "PCB草图" plane through (0, 3.8, 0) normal (0, 1, 0) x (-1, 0, 0)
  line L0 (96, -90.5) -> (87, -90.5)
  line L1 (87, -90.5) -> (87, -107.6002)
  line L2 (49.4998, -147) -> (-55.0478, -147)
  line L3 (-54.9998, -147) -> (-54.9998, 147)
  line L4 (-55.0478, 147) -> (87, 147)
  line L5 (87, 147) -> (87, 14)
  line L6 (87, 14) -> (96, 14)
  line L7 (96, -14) -> (96, 14)
  line L8 (87, -14) -> (96, -14)
  line L9 (87, -14) -> (87, -62.5)
  line L10 (87, -62.5) -> (96, -62.5)
  line L11 (96, -62.5) -> (96, -90.5)
  line L12 (87, -107.6002) -> (49.4998, -107.6002)
  line L13 (49.4998, -107.6002) -> (49.4998, -147)
  constraints: 28 end point, 2 point on line
sketch "草图3" plane through (0, 0, 0) normal (1, 0, 0) x (0, 1, 0)
  line L0 (0, 0) -> (3.5, 0)
  line L1 (3.5, 0) -> (3.5, 4)
  line L2 (3.5, 4) -> (0, 4)
  line L3 (0, 4) -> (0, 0)
  line L4 (3.5, 4) -> (8.8, 4)
  line L5 (8.8, 4) -> (8.8, 0)
  line L6 (8.8, 0) -> (3.5, 0)
  line L7 (3.5, 0) -> (3.5, 4)
  line L8 (0, 0) -> (3, 0)
  line L9 (3, 0) -> (3, -4)
  line L10 (3, -4) -> (0, -4)
  line L11 (0, -4) -> (0, 0)
  line L12 (3, -4) -> (7, -4)
  line L13 (7, -4) -> (7, 0)
  line L14 (7, 0) -> (3, 0)
  line L15 (3, 0) -> (3, -4)
  line L16 (7, -4) -> (10, -4)
  line L17 (10, -4) -> (10, 0)
  line L18 (10, 0) -> (7, 0)
  line L19 (7, 0) -> (7, -4)
  line L20 (3, -4) -> (1.8, -4)
  line L21 (1.8, -4) -> (1.8, 11)
  line L22 (1.8, 11) -> (3, 11)
  line L23 (3, 11) -> (3, -4)
  line L24 (3, -4) -> (6, -4)
  line L25 (6, -4) -> (6, -8.0299)
  line L26 (6, -8.0299) -> (3, -8.0299)
  line L27 (3, -8.0299) -> (3, -4)
  line L28 (6, -4) -> (5, -4)
  line L29 (5, -4) -> (5, 11)
  line L30 (5, 11) -> (6, 11)
  line L31 (6, 11) -> (6, -4)
  dimension "d23" = 3.5
  dimension "d24" = 4
  dimension "d25" = 5.3
  dimension "d26" = 4
  dimension "d27" = 3
  dimension "d28" = 4
  dimension "d29" = 4
  dimension "d30" = 4
  dimension "d31" = 3
  dimension "d32" = 4
  dimension "d33" = 1.2
  dimension "d34" = 15
  dimension "d35" = 3
  dimension "d36" = 1
  dimension "d37" = 15
  constraints: 64 end point
  measures "d23" distance of L2.end L1.end
  measures "d24" distance of L1.end L0.end
  measures "d25" distance of L5.end L6.end
  measures "d26" distance of L4.end L5.end
  measures "d27" distance of L9.end L10.end
  measures "d28" distance of L8.end L9.end
  measures "d29" distance of L14.end L13.end
  measures "d30" distance of L13.end L12.end
  measures "d31" distance of L18.end L17.end
  measures "d32" distance of L17.end L16.end
  measures "d33" distance of L21.end L22.end
  measures "d34" distance of L20.end L21.end
  measures "d35" distance of L25.end L26.end
  measures "d36" distance of L29.end L30.end
  measures "d37" distance of L28.end L29.end
extrude "BottomPlate拉伸" add sketch "BottomPlate草图" along normal blind 2 contours A4 L3 A7 L2 A6 L1 A5 L0 | A0 | A1 | A2 | A3 | A8 | A9 | A10 | A11 | A12 | A13 | A14 | A15 | A16 | A17 | A18 | A19 | A20 | A21 | A22 | A23 | A24 | A25 | A26 | A27 | A28 | A29
extrude "FloorFirst拉伸" add sketch "FloorFirst草图" along normal blind 3 separate body contours L0 A1 L1 A2 L2 A3 L3 A0
extrude "FloorSecond拉伸" add sketch "FloorSecond草图" along normal blind 4 separate body
extrude "TopPlate拉伸" add sketch "TopPlate草图" along normal blind 3 separate body contours L2 A1 L3 A2 L4 A3 L1 A0 L0 | A4 | A5 | A6 | A7 | A21 | L41 L52 A39 L51 L38 | L51 A39 L52 L41 L42 L49 L46 L47 L48 L44 L56 A40 L55 L40 L63 A41 L64 L39 L60 A42 L59 L38 | L59 A42 L60 L39 L38 | A39 L52 L51 | L51 L52 A39 | L41 L44 L43 L42 | A42 L60 L59 | L59 L60 A42 | L41 L40 L55 A40 L56 | L64 A41 L63 L40 L39 | A40 L55 L56 | L56 L55 A40 | A41 L63 L64 | L64 L63 A41 | A44 | A46 | A48 | A50 | A51
extrude "拉伸5" add sketch "PCB草图" along normal blind 1.2 separate body
extrude "拉伸6" add sketch "PositionPlate草图" along normal blind 1 separate body
hole "底板固定孔" at (-92, 0, -152) at (-94, 0, -103.25) at (-94, 0, -49.75) at (-94, 0, -26.75) at (-94, 0, 26.75) at (-92, 0, 152) at (0, 0, 154) at (92, 0, 152) at (94, 0, 0) at (92, 0, -152) at (0, 0, -153.5) direction (0, 1, 0) diameter 3.2 end through all counterbore diameter 6.2 counterbore depth 1 bodies 1
hole "底板PCB定位孔" at (-75, 0, -55) at (-91.5, 0, -87.5) at (-91.5, 0, -65.5) at (-91.5, 0, -11) at (-91.5, 0, 11) at (-75, 0, 55) at (-16, 0, -55) at (-16, 0, 55) at (-57.5, 0, 120) at (43, 0, -55) at (43, 0, 55) at (-82.4998, 0, -142.4002) at (-82.4998, 0, -112.2002) at (-53.9998, 0, -112.2002) at (-53.9998, 0, -142.4002) direction (0, 1, 0) diameter 2.7 end through all counterbore diameter 5.2 counterbore depth 1 bodies 1 5 6
sketch "草图8" plane through (0, 12, 0) normal (0, 1, 0) x (1, 0, 0)
  circle A0 centre (-92, -152) radius 1.6 projected
  circle A1 centre (-94, -26.75) radius 1.6 projected
  circle A2 centre (-94, 26.75) radius 1.6 projected
  circle A3 centre (-92, 152) radius 1.6 projected
  circle A4 centre (0, 153.5) radius 1.6 projected
  circle A5 centre (92, 152) radius 1.6 projected
  circle A6 centre (94, 0) radius 1.6 projected
  circle A7 centre (92, -152) radius 1.6 projected
  circle A8 centre (0, -154) radius 1.6 projected
  point P0 (0, 0)
hole "顶部面板定位孔" at (-92, 12, 152) at (0, 12, 154) at (92, 12, 152) at (94, 12, 0) at (92, 12, -152) at (0, 12, -153.5) at (-92, 12, -152) at (-94, 12, -26.75) at (-94, 12, 26.75) direction (0, -1, 0) diameter 3.2 end through all counterbore diameter 6.2 counterbore depth 1 bodies 4
